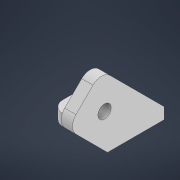
# Autodesk Inventor part: 45 degree inside angle bracket
Saved by Autodesk Inventor 2022 (Build 260153000, 153)
## iProperties
Created: 2022-01-18
Part Number: 45 degree inside angle bracket
Material: Generic
Document SubType Name: Modeling
Designer: izack
Density: 1 g/cm^3
Appearance: Default
Author: izack
## iProperties of the stored document 45 degree inside angle bracket_3DPrint.ipt
Created: 2022-01-18
Part Number: 45 degree inside angle bracket_3DPrint
Material: Generic
Document SubType Name: Modeling
Designer: izack
Density: 1 g/cm^3
Appearance: Default
Author: izack
Autodesk Inventor part; units mm, degrees
ref_plane "YZ Plane" through (0, 0, 0) normal (1, 0, 0) x (0, 1, 0)
ref_plane "XZ Plane" through (0, 0, 0) normal (0, 1, 0) x (-1, 0, 0)
ref_plane "XY Plane" through (0, 0, 0) normal (0, 0, 1) x (1, 0, 0)
sketch "Sketch1" plane through (0, 0, 0) normal (0, 1, 0) x (-1, 0, 0)
  line L0 (0, 0) -> (15, 0)
  line L1 (15, 0) -> (15, -15)
  line L2 (15, -15) -> (0, -15)
  line L3 (0, -15) -> (0, 0)
  circle A0 centre (7.5, -7.5) radius 1.75
  dimension "d0" = 15
  dimension "d1" = 15
  dimension "d2" = 3.5
  constraints: 8 end point, 2 parallel, 1 centre point, 1 horizontal, 1 perpendicular
  measures "d0" distance of L1.end L2.end
  measures "d1" distance of L0.end L1.end
  measures "d2" diameter of A0
extrude "Extrusion1" add sketch "Sketch1" along normal blind 3
sketch "Sketch2" plane through (0, 0, 0) normal (1, 0, 0) x (0, 0, -1)
  line L0 (15, 0) -> (0, 0) projected
  line L1 (0, 0) -> (-10.6066, 10.6066)
  line L2 (0, 0) -> (15, 0) construction
  line L3 (15, 0) -> (40.6066, 0) construction
  line L4 (-3.1066, 18.1066) -> (-10.6066, 10.6066)
  line L5 (15, 3) -> (0, 3) projected
  line L6 (15, 3) -> (-1.6066, 19.6066)
  line L7 (15, 3) -> (38.4853, 3) construction
  line L8 (-1.6066, 19.6066) -> (-3.1066, 18.1066)
  line L9 (-1.6066, 19.6066) -> (-10.6066, 10.6066) construction
  line L10 (-6.1066, 15.1066) -> (7.5, 1.5) construction
  circle A0 centre (-0.8033, 9.8033) radius 1.75
  line L11 (15, 3) -> (15, 0)
  line L12 (0, 0) -> (15, 0)
  line L13 (15, 3) -> (-1.6066, 19.6066)
  line L14 (-1.6066, 19.6066) -> (-10.6066, 10.6066)
  line L15 (-10.6066, 10.6066) -> (0, 0)
  dimension "d5" = 15
  dimension "d6" = 135
  dimension "d10" = 135
  dimension "d12" = 3.5
  dimension "d13" = 7.5
  constraints: 28 end point, 3 horizontal, 3 perpendicular, 2 equal length, 2 point on line, 1 centre point, 1 collinear, 1 midpoint
  measures "d5" distance of L0.end L1.end
  measures "d6" angle of L2 L1
  measures "d10" angle of L7 L6
  measures "d12" diameter of A0
  measures "d13" distance from line of L4 A0.centre
extrude "Extrusion3" add sketch "Sketch2" against normal blind 3
fillet "Fillet1" radius 3.175 4 edges at (-15, 1.5, -15) (-15, 1.5, 0) (-1.5, 19.6066, 1.6066) (-1.5, 10.6066, 10.6066)
fillet "Fillet2" radius 3.175 2 edges at (-3, 3, -7.5) (-3, 1.5, 0)
body "Solid1"
